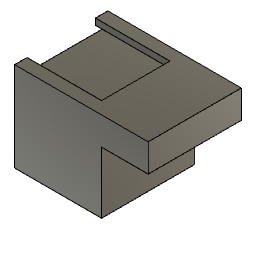
Support Tasseaux (Autodesk Fusion 360 design; units mm, degrees)
Autodesk Fusion 360 part; units mm, degrees
sketch "Esquisse1" plane through (0, 0, 0) normal (0, 0, 1) x (1, 0, 0)
  line L0 (0, 0) -> (0, 15)
  line L1 (0, 15) -> (-14, 15)
  line L2 (-14, 15) -> (-14, 0)
  line L3 (-14, 0) -> (0, 0)
  dimension "d1" = 90
  dimension "d3" = 14
  dimension "d15" = 15
  constraint coincident L0.start L3.end
  constraint vertical L0
  constraint parallel L0 L2
  measures "d1" angle of L0 L1
  measures "d3" distance of L0.end L1.end
  measures "d15" distance of L1 L3
extrude "Extrusion1" add sketch "Esquisse1" along normal blind 1.2 makes body 1
sketch "Esquisse3" plane through (0, 0, 1.2) normal (0, 0, 1) x (-1, 0, 0)
  line L0 (14, 0) -> (0, 0)
  line L1 (0, 0) -> (0, -15)
  line L2 (0, -15) -> (14, -15)
  line L3 (14, -15) -> (14, 0)
  line L4 (14, -15) -> (0, -15)
  line L5 (0, 0) -> (14, 0)
  line L6 (14, -2) -> (2, -2)
  line L7 (2, -2) -> (2, -13)
  line L8 (2, -13) -> (14, -13)
  line L9 (14, -15) -> (14, -13)
  line L10 (14, -2) -> (14, 0)
  line L11 (0, -15) -> (0, 0)
  dimension "d14" = 2
  dimension "d16" = 11
  dimension "d17" = 2
  constraint coincident L2.end L3.start
  constraint coincident L1.end L2.start
  constraint coincident L0.end L1.start
  constraint coincident L0.start L3.end
  constraint coincident L3 L6.start
  constraint parallel L0 L6
  constraint parallel L3 L7
  constraint coincident L3 L8.end
  constraint parallel L0 L8
  constraint parallel L3 L9
  constraint parallel L3 L10
  measures "d14" distance of L5 L6
  measures "d16" distance of L6 L8
  measures "d17" distance of L7 L11
extrude "Extrusion2" add sketch "Esquisse3" along normal blind 11 contours L0 L1 L2 L3 L4 L5 L6 L7 L8 L9 L10 L11 bodies 1
sketch "Esquisse4" plane through (0, 0, 12.2) normal (0, 0, 1) x (-1, 0, 0)
  line L0 (14, -15) -> (14, -13)
  line L1 (14, -13) -> (2, -13)
  line L2 (2, -13) -> (2, -2)
  line L3 (2, -2) -> (14, -2)
  line L4 (14, -2) -> (14, 0)
  line L5 (14, 0) -> (0, 0)
  line L6 (0, 0) -> (0, -15)
  line L7 (0, -15) -> (14, -15)
  line L8 (14, -1) -> (14, 0)
  line L9 (0, 0) -> (14, 0)
  line L10 (0, 0) -> (0, -15)
  line L11 (0, -15) -> (14, -15)
  line L12 (14, -15) -> (14, -14)
  line L13 (14, -14) -> (2, -14)
  line L14 (2, -14) -> (2, -1)
  line L15 (2, -1) -> (14, -1)
  dimension "d18" = 2
  constraint midpoint L4 L8.start
  constraint coincident L4.end L5.start
  constraint coincident L5.end L6.start
  constraint coincident L6.end L7.start
  constraint coincident L0.start L7.end
  constraint midpoint L0 L12.end
  constraint parallel L7 L13
  constraint parallel L10 L14
  constraint parallel L9 L15
  measures "d18" distance of L10 L14
extrude "Extrusion3" add sketch "Esquisse4" along normal blind 1.2 contours L0 L2 L4 L5 L6 L7 L8 L9 L10 L11 L12 L13 L14 L15 bodies 1
sketch "Esquisse5" plane through (0, 0, 13.4) normal (0, 0, 1) x (-1, 0, 0)
  line L0 (0, 0) -> (0, -15)
  line L1 (0, -15) -> (14, -15)
  line L2 (14, -15) -> (14, -14)
  line L3 (14, -14) -> (2, -14)
  line L4 (2, -14) -> (2, -1)
  line L5 (2, -1) -> (14, -1)
  line L6 (14, -1) -> (14, 0)
  line L7 (14, 0) -> (0, 0)
  line L8 (14, -15) -> (0, -15)
  line L9 (0, -15) -> (0, 0)
  line L10 (0, 0) -> (14, 0)
  line L11 (14, 0) -> (14, -2)
  line L12 (14, -15) -> (14, -13)
  line L13 (14, -13) -> (2, -13)
  line L14 (2, -13) -> (2, -2)
  line L15 (2, -2) -> (14, -2)
  dimension "d23" = 2
  dimension "d24" = 2
  dimension "d25" = 2
  constraint coincident L1.end L2.start
  constraint coincident L0.end L1.start
  constraint coincident L0.start L7.end
  constraint coincident L6.end L7.start
  constraint parallel L6 L11
  constraint parallel L2 L12
  constraint vertical L14
  constraint parallel L8 L13
  constraint parallel L10 L15
  measures "d23" distance of L9 L14
  measures "d24" distance of L8 L13
  measures "d25" distance of L10 L15
extrude "Extrusion4" add sketch "Esquisse5" along normal blind 1 bodies 1
fillet "Congé1" radius 1.5 2 edges at (-14, 13.5, 12.2) (-14, 1.5, 12.2) on bodies 1
sketch "Esquisse7" plane through (0, 0, 14.4) normal (0, 0, 1) x (-1, 0, 0)
  line L0 (14, -15) -> (14, -13)
  line L1 (14, -13) -> (2, -13)
  line L2 (2, -13) -> (2, -2)
  line L3 (2, -2) -> (14, -2)
  line L4 (14, -2) -> (14, 0)
  line L5 (14, 0) -> (0, 0)
  line L6 (0, 0) -> (0, -15)
  line L7 (0, -15) -> (14, -15)
  line L8 (-7.5, -15) -> (-7.5, 0)
  line L9 (-7.5, 0) -> (0, 0)
  line L10 (0, 0) -> (0, -15)
  line L11 (0, -15) -> (-7.5, -15)
  dimension "d44" = 7.5
  constraint parallel L6 L8
  constraint coincident L5.end L6.start
  constraint coincident L6.end L7.start
  constraint horizontal L8.end L5.end
  constraint horizontal L6.end L8.start
  measures "d44" distance of L8 L10
extrude "Extrusion6" add sketch "Esquisse7" against normal blind 4.5 contours L6 L8 L9 L10 L11 bodies 1
sketch "Esquisse8" plane through (0, 0, 12.2) normal (0, 0, 1) x (-1, 0, 0)
  line L0 (12.5, -14) -> (12.5, -13)
  line L1 (12.5, -13) -> (2, -13)
  line L2 (2, -13) -> (2, -14)
  line L3 (2, -14) -> (12.5, -14)
  line L4 (13, -14) -> (2, -14)
  line L5 (2, -1.4) -> (2, -14)
  line L6 (2, -1.4) -> (13, -1.4)
  line L7 (13, -1.4) -> (13, -14)
  line L8 (-7.5, -15) -> (14, -15)
  dimension "d38" = 12.6
  dimension "d39" = 11
  constraint coincident L2.end L3.start
  constraint parallel L2 L5
  constraint parallel L1 L6
  constraint parallel L5 L7
  constraint parallel L4 L8
  measures "d38" distance of L0.start L6
  measures "d39" distance of L4.start L2.end
extrude "Extrusion7" add sketch "Esquisse8" along normal blind 1.1 separate body makes body 2
equation "d1 = Angle"
equation "d3 = Longueur_Support + 2 * Epaisseur_Support"
equation "d14 = Epaisseur_Support"
equation "d15 = Largeur_Tasseau + 2 * Epaisseur_Support"
equation "d16 = Largeur_Tasseau"
equation "d17 = Epaisseur_Support"
equation "d18 = Epaisseur_Support"
equation "d38 = Largeur_Tasseau + Epaisseur_Support - 0.4 mm"
equation "d39 = Longueur_Support + 1 mm"
equation "Angle = 90 deg"
equation "Longueur_Support = 10 mm"
equation "Epaisseur_Support = 2 mm"
equation "Largeur_Tasseau = 11 mm"
equation "Hauteur_Tasseau = 11 mm"
named bodies: "Support", "Cache"
